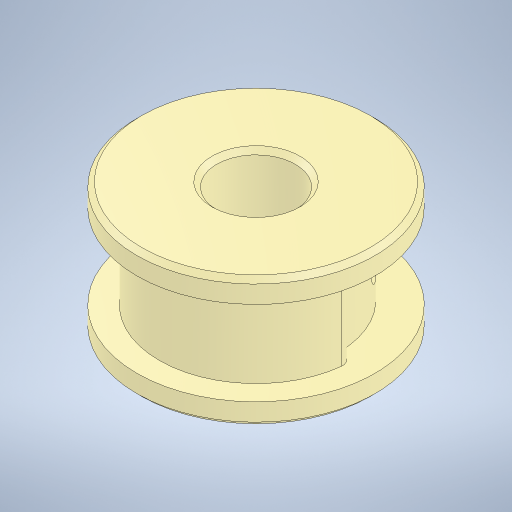
# Autodesk Inventor part: Spring Spool
Saved by Autodesk Inventor 2023.4 (Build 274418000, 418)
## iProperties
Created: 2024-03-24
Part Number: Spring Spool
Material: Nylon 6/6
Document SubType Name: Modeling
Designer: Nathan Cai
Density: 1.13 g/cm^3
Appearance: Nylon 6
Author: Nathan Cai
Autodesk Inventor part; units mm, degrees
ref_plane "XZ Plane" through (0, 0, 0) normal (0, 1, 0) x (-1, 0, 0)
sketch "Sketch1" plane through (0, 0, 0) normal (1, 0, 0) x (0, 1, 0)
  line L0 (0, 0) -> (13.7625, 0)
  line L1 (13.7625, 0) -> (13.7625, 10.31875)
  line L2 (13.7625, 10.31875) -> (0, 10.31875)
  line L3 (0, 10.31875) -> (0, 0)
  line L4 (13.7625, 10.31875) -> (11.38125, 10.31875)
  line L5 (11.38125, 10.31875) -> (11.38125, 12.7)
  line L6 (11.38125, 12.7) -> (13.7625, 12.7)
  line L7 (13.7625, 12.7) -> (13.7625, 10.31875)
  line L8 (0, 10.31875) -> (2.38125, 10.31875)
  line L9 (2.38125, 10.31875) -> (2.38125, 12.7)
  line L10 (2.38125, 12.7) -> (0, 12.7)
  line L11 (0, 12.7) -> (0, 10.31875)
  line L12 (13.7625, 4.2) -> (0, 4.2)
  line L13 (0, 4.2) -> (0, 0)
  line L14 (0, 0) -> (13.7625, 0)
  line L15 (13.7625, 0) -> (13.7625, 4.2)
  point P0 (0, 4.2)
  dimension "d1" = 10.31875
  dimension "d2" = 2.38125
  dimension "d3" = 2.38125
  dimension "d4" = 12.7
  dimension "d5" = 4.2
  dimension "d29" = 9
  constraints: 32 end point, 8 parallel, 4 horizontal, 4 perpendicular, 2 point on line
  measures "d1" distance of L1.end L0.end
  measures "d2" distance of L5.end L6.end
  measures "d3" distance of L10.end L9.end
  measures "d4" distance between parallel lines of L0 L6
  measures "d5" distance between parallel lines of L0 L12
  measures "d29" distance between parallel lines of L9 L5
revolve "Revolution1" add sketch "Sketch1" angle 360 about axis through (0, 0, 0) along (0, 1, 0) contours L3 L2 L1 L12 | L11 L10 L9 L2 | L2 L5 L6 L7
sketch "Sketch2" plane through (0, 2.38125, 0) normal (0, 1, 0) x (1, 0, 0)
  circle A0 centre (0, 0) radius 4.2
  circle A1 centre (0, 0) radius 6.2
  line L0 (4.2, 0) -> (6.2, 0)
  line L1 (0, 4.2) -> (0, 6.2)
  circle A2 centre (0, 0) radius 10.31875
  line L2 (0, 6.2) -> (-9.425317, 6.2)
  line L3 (-9.425317, 6.2) -> (-9.425317, 4.2)
  line L4 (-9.425317, 4.2) -> (0, 4.2)
  line L5 (0, 4.2) -> (0, 6.2)
  line L6 (10.31875, 0) -> (8.81875, 0)
  arc A3 (8.81875, 0) -> (-10.31875, 0) centre (-0.75, 0) ccw
  dimension "d7" = 2
  dimension "d30" = 1.5
  constraints: 14 end point, 9 point on circle, 4 point on line, 3 horizontal, 2 centre point, 2 parallel, 2 perpendicular, 1 line through centre, 1 tangent
  measures "d7" radial gap between concentric circles of A0 A1
  measures "d30" distance of L6.start L6.end
sketch "Sketch2 outline for Extrusion1" plane through (0, 2.38125, 0) normal (0, 1, 0) x (1, 0, 0)
  arc A0 (-10.31875, 0) -> (8.81875, 0) centre (-0.75, 0) cw
  arc A1 (10.31875, 0) -> (-10.31875, 0) centre (0, 0) ccw
  line L0 (8.81875, 0) -> (10.31875, 0)
extrude "Extrusion1" cut sketch "Sketch2 outline for Extrusion1" along normal up to surface (9 mm away)
ref_plane "Work Plane1" through (0, 0, 0) normal (-0.7071068, 0, 0.7071068) x (0, -1, 0)
sketch "Sketch3" plane through (0, 0, 0) normal (-0.7071068, 0, 0.7071068) x (0, -1, 0)
  line L0 (0, 0) -> (-13.7625, 0) construction
  line L1 (-13.7625, 4.2) -> (-13.7625, -4.2)
  circle A0 centre (-6.88125, 0) radius 1.651
  dimension "d12" = 3.302
  constraints: 2 end point, 2 midpoint, 1 centre point
  measures "d12" diameter of A0
extrude "Extrusion2" cut sketch "Sketch3" against normal through all
chamfer "Chamfer1" distance 0.5 angle 45 2 edges at (0, 0, -4.2) (0, 13.7625, -4.2)
chamfer "Chamfer2" distance 0.5 angle 45 1 edges at (6.7558, 8.4269, -5.935)
chamfer "Chamfer3" distance 0.5 angle 45 2 edges at (0, 13.7625, -12.7) (0, 0, -12.7)
fillet "Fillet3" radius 1 1 edges at (10.3188, 6.8812, 0)
equation "\"d3\" = d2"
body "Solid1"
